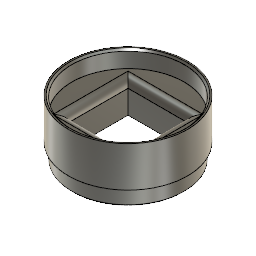
mid v8 (Autodesk Fusion 360 design; units mm, degrees)
Autodesk Fusion 360 part; units mm, degrees
sketch "Sketch1" plane through (0, 0, 0) normal (0, 0, 1) x (1, 0, 0)
  circle A0 centre (0, 0) radius 35.5
  dimension "d1" = 71
  measures "d1" diameter of A0
extrude "Extrude1" add sketch "Sketch1" along normal blind 34
sketch "Sketch2" plane through (0, 0, 34) normal (0, 0, 1) x (-1, 0, 0)
  circle A0 centre (0, 0) radius 35.5
  circle A1 centre (0, 0) radius 33.5
  dimension "d6" = 67
  measures "d6" diameter of A1
extrude "Extrude2" cut sketch "Sketch2" against normal blind 10 contours A1
sketch "Sketch3" plane through (0, 0, 0) normal (0, 0, -1) x (1, 0, 0)
  circle A0 centre (0, 0) radius 35.5
  line L0 (22.5, 22.5) -> (-22.5, 22.5)
  line L1 (-22.5, 22.5) -> (-22.5, -22.5)
  line L2 (-22.5, -22.5) -> (22.5, -22.5)
  line L3 (22.5, -22.5) -> (22.5, 22.5)
  line L4 (22.5, 22.5) -> (-22.5, -22.5) construction
  line L5 (-22.5, 22.5) -> (22.5, -22.5) construction
  dimension "d9" = 45
extrude "Extrude3" cut sketch "Sketch3" against normal blind 20 contours L0 L1 L2 L3
sketch "Sketch4" plane through (0, 0, 24) normal (0, 0, 1) x (-1, 0, 0)
  circle A0 centre (0, 0) radius 33.5
  line L0 (-17.5, -17.5) -> (17.5, -17.5)
  line L1 (17.5, -17.5) -> (17.5, 17.5)
  line L2 (17.5, 17.5) -> (-17.5, 17.5)
  line L3 (-17.5, 17.5) -> (-17.5, -17.5)
  line L4 (-17.5, -17.5) -> (17.5, 17.5) construction
  line L5 (17.5, -17.5) -> (-17.5, 17.5) construction
  dimension "d12" = 35
extrude "Extrude4" cut sketch "Sketch4" against normal blind 10 contours L0 L1 L2 L3
sketch "Sketch5" plane through (0, 0, 0) normal (0, 0, -1) x (1, 0, 0)
  line L0 (-22.5, 22.5) -> (22.5, 22.5)
  line L1 (22.5, 22.5) -> (22.5, -22.5)
  line L2 (22.5, -22.5) -> (-22.5, -22.5)
  line L3 (-22.5, -22.5) -> (-22.5, 22.5)
  circle A0 centre (0, 0) radius 35.5
  circle A1 centre (0, 0) radius 33.5
  circle A2 centre (0, 0) radius 35.5
  dimension "d16" = 2
  measures "d16" distance of A0 A1
extrude "Extrude5" cut sketch "Sketch5" against normal blind 10 contours A0 A2
chamfer "Chamfer2" distance 1 angle 45 6 edges at (31.233, -12.1141, 34) (-31.233, 12.1141, 0) (0, 22.5, 0) (22.5, 0, 0) (0, -22.5, 0) (-22.5, 0, 0)
fillet "Fillet1" radius 5 4 edges at (0, 17.5, 24) (-17.5, 0, 24) (0, -17.5, 24) (17.5, 0, 24)
